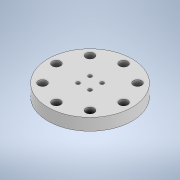
# Autodesk Inventor part: Forma-kolo_dol
Saved by Autodesk Inventor 2020 (Build 240168000, 168)
## iProperties
Created: 2023-02-02
Part Number: Forma-kolo_dol
Material: Ogólny
Document SubType Name: Modeling
Designer: User
Density: 1 g/cm^3
Appearance: Domyślna
Author: User
Autodesk Inventor part; units mm, degrees
ref_plane "YZ Plane" through (0, 0, 0) normal (1, 0, 0) x (0, 1, 0)
ref_plane "XZ Plane" through (0, 0, 0) normal (0, 1, 0) x (-1, 0, 0)
ref_plane "XY Plane" through (0, 0, 0) normal (0, 0, 1) x (1, 0, 0)
sketch "Szkic1" plane through (0, 0, 0) normal (0, 1, 0) x (-1, 0, 0)
  circle A0 centre (0, 0) radius 10
  circle A1 centre (0, 0) radius 17.5
  line L0 (0, 17.5) -> (0, -17.5)
  line L1 (-17.5, 0) -> (17.5, 0)
  circle A2 centre (2.5, 2.5) radius 0.75
  circle A3 centre (2.5, -2.5) radius 0.75
  circle A4 centre (-2.5, 2.5) radius 0.75
  circle A5 centre (-2.5, -2.5) radius 0.75
  circle A6 centre (0, 14) radius 1.75
  circle A7 centre (0, -14) radius 1.75
  circle A8 centre (14, 0) radius 1.75
  circle A9 centre (-14, 0) radius 1.75
  line L2 (-2.5, -2.5) -> (-12.3744, -12.3744)
  line L3 (2.5, 2.5) -> (12.3744, 12.3744)
  line L4 (2.5, -2.5) -> (12.3744, -12.3744)
  line L5 (-2.5, 2.5) -> (-12.3744, 12.3744)
  circle A10 centre (9.8995, 9.8995) radius 1.75
  circle A11 centre (-9.8995, -9.8995) radius 1.75
  line L6 (-2.5, 2.5) -> (2.5, -2.5)
  line L7 (2.5, 2.5) -> (-2.5, -2.5)
  circle A12 centre (-9.8995, 9.8995) radius 1.75
  circle A13 centre (9.8995, -9.8995) radius 1.75
  dimension "d1" = 35
  dimension "d0" = 20
  dimension "d2" = 1.5
  dimension "d3" = 5
  dimension "d4" = 5
  dimension "d5" = 28
  dimension "d6" = 3.5
  dimension "d7" = 28
  dimension "d8" = 3.5
  dimension "d9" = 3.5
  dimension "d11" = 19.799
  constraints: 16 end point, 13 centre point, 8 point on line, 2 coincident, 1 collinear, 1 perpendicular, 18 other
  measures "d0" diameter of A0
  measures "d2" diameter of A2
  measures "d3" distance of L4.start L3.start
  measures "d4" distance of L5.start L3.start
  measures "d5" distance of A7.centre A6.centre
  measures "d6" diameter of A6
  measures "d7" distance of A9.centre A8.centre
  measures "d8" diameter of A8
  measures "d9" diameter of A10
  measures "d11" horizontal distance of A11.centre A10.centre
extrude "Wyciągnięcie proste1" add sketch "Szkic1" along normal blind 5 contours L1 L7 A2 L3 A0 | L1 A8 A1 L4 A13 A0 | A0 L4 A3 L6 L1 | A0 L3 A10 A1 L1 A8 | L3 A2 L7 L0 A0 | A0 L0 A6 A1 L3 A10 | L4 A13 A1 L0 A7 A0 | A0 L0 L6 A3 L4 | L6 A4 L5 A0 L0 | L7 A5 L2 A0 L1 | L1 A0 L5 A4 L6 | L0 A0 L2 A5 L7 | A0 L5 A12 A1 L0 A6 | L0 A7 A1 L2 A11 A0 | L1 A9 A1 L5 A12 A0 | A0 L2 A11 A1 L1 A9
